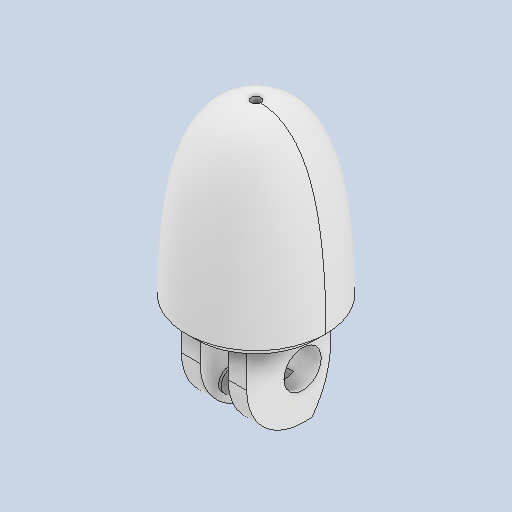
# Autodesk Inventor part: Lil_3
Saved by Autodesk Inventor 2022 (Build 260153000, 153)
## iProperties
Created: 2023-01-15
Part Number: Lil_3
Material: ABS Plastic
Document SubType Name: Modeling
Designer: 48735
Density: 1.06 g/cm^3
Appearance: Smooth - White
Author: 48735
Autodesk Inventor part; units mm, degrees
ref_plane "YZ Plane" through (0, 0, 0) normal (1, 0, 0) x (0, 1, 0)
ref_plane "XZ Plane" through (0, 0, 0) normal (0, 1, 0) x (-1, 0, 0)
sketch "Sketch1" plane through (0, 0, 0) normal (0, 1, 0) x (-1, 0, 0)
  circle A0 centre (0, 0) radius 7.5
  line L0 (3.5, 0) -> (3.5, -4.5)
  line L1 (3.5, -4.5) -> (1.5, -4.5)
  line L2 (1.5, -2.5) -> (1.5, 0)
  line L3 (3.5, 0) -> (3.5, 4.5)
  line L4 (3.5, 4.5) -> (1.5, 4.5)
  line L5 (1.5, 4.5) -> (1.5, 0)
  line L6 (-1.5, 0) -> (-1.5, 4.5)
  line L7 (-1.5, 4.5) -> (-3.5, 4.5)
  line L8 (-3.5, 4.5) -> (-3.5, 0)
  line L9 (-3.5, -4.5) -> (-3.5, 0)
  line L10 (-3.5, -4.5) -> (-1.5, -4.5)
  line L11 (-1.5, -2.5) -> (-1.5, 0)
  line L12 (3.5, -4.5) -> (3.5, -2.5)
  line L13 (1.5, -2.5) -> (-1.5, -2.5)
  line L14 (-3.5, -4.5) -> (3.5, -4.5)
  constraints: 30 end point, 7 perpendicular, 5 point on line, 3 collinear, 1 centre point, 1 coincident, 1 parallel, 1 vertical
extrude "Extrusion1" add sketch "Sketch1" along normal blind 10 contours L0 L1 L14 L10 L9 L8 L7 L6 L11 L13 L2 L5 L4 L3
fillet "Fillet1" radius 6 2 edges at (2.5, 0, 4.5) (-2.5, 0, 4.5)
fillet "Fillet2" radius 10 3 edges at (-2.5, 0, -4.5) (0, 0, -4.5) (2.5, 0, -4.5)
sketch "Sketch2" plane through (0, 10, 0) normal (0, 1, 0) x (1, 0, 0)
  circle A0 centre (0, 0) radius 7.5
  circle A1 centre (0, 0) radius 1.25
  dimension "d12" = 15
  dimension "d13" = 2.5
  constraints: 2 centre point, 2 coincident
  measures "d12" diameter of A0
  measures "d13" diameter of A1
extrude "Extrusion2" add sketch "Sketch2" along normal blind 1
chamfer "Chamfer1" distance 1 angle 45 1 edges at (-7.5, 10, 0)
fillet "Fillet3" radius 0.25 1 edges at (-1.25, 10, 0)
sketch "Sketch3" plane through (3.5, 0, -1.5) normal (1, 0, 0) x (0, 0, -1)
  line L0 (0, 0) -> (0, 5)
  point P0 (-1.5, 0)
  dimension "d20" = 5
  constraints: 2 end point, 1 vertical
  measures "d20" distance of L0.start L0.end
hole "Hole1" at (3.5, 5, -1.5) direction (-1, 0, 0) diameter 4 depth 10
sketch "Sketch4" plane through (1.5, 0, -2.5) normal (-1, 0, 0) x (0, 0, 1)
  line L0 (7, 6) -> (7, 10) projected
  circle A0 centre (3.75, 3) radius 1.25
  point P0 (2.5, 0)
  constraints: 1 centre point
extrude "Extrusion3" add sketch "Sketch4" along normal blind 1.5
chamfer "Chamfer2" distance 0.25 distance2 1.25 1 edges at (0, 3, 0) measured on face at (0, 3, 0.5)
sketch "Sketch5" plane through (-1.5, 0, -1.5) normal (1, 0, 0) x (0, 0, -1)
  circle A0 centre (-2.75, 3) radius 1.25 projected
  circle A1 centre (-2.75, 3) radius 1.25
  point P0 (-1.5, 0)
  constraints: 1 centre point, 1 coincident
extrude "Extrusion4" add sketch "Sketch5" along normal blind 1.5
chamfer "Chamfer3" distance 0.25 distance2 1.25 1 edges at (0, 3, 2.5) measured on face at (0, 3, 2.4)
ref_plane "Work Plane1" through (-1.25, 11, 0) normal (0, 0, 1) x (1, 0, 0)
sketch "Sketch12" plane through (-1.25, 11, 0) normal (0, 0, 1) x (1, 0, 0)
  line L0 (8.75, 0) -> (-6.25, 0) projected
  line L1 (1.25, 0) -> (8.75, 0)
  line L2 (1.25, 0) -> (1.25, 18)
  line L3 (1.25, 18) -> (1.25, 20.598)
  line L4 (1.25, 18) -> (5, 18) construction
  line L5 (5, 18) -> (8.75, 15.5074) construction
  line L6 (8.75, 15.5074) -> (8.75, 0) construction
  spline S0 degree 3 poles (1.25, 18) (5, 18) (8.75, 15.5074) (8.75, 0) knots 1 1 1 1 2 2 2 2
  point P0 (1.25, -11)
  dimension "d63" = 18
  constraints: 6 end point, 2 perpendicular, 1 collinear, 1 midpoint, 1 point on line, 1 vertical, 3 other
  measures "d63" distance of L1.start L2.end
revolve "Revolution1" add sketch "Sketch12" angle 360 about axis through (0, 11, 0) along (0, 1, 0)
sketch "Sketch13" plane through (0, 11, 0) normal (0, -1, 0) x (1, 0, 0)
  circle A0 centre (0, 0) radius 0.5
  dimension "d65" = 1
  constraints: 1 centre point, 1 coincident
  measures "d65" diameter of A0
extrude "Extrusion11" cut sketch "Sketch13" against normal blind 22.7
fillet "Fillet4" radius 0.75 1 edges at (-0.5, 11, 0)
body "Solid1"
